Autodesk Fusion 360 part; units mm, degrees
note: some values were not read from the file. Set by a fixed rule: which sketch regions a step uses.
(part 9 of 10)
  spline S50 degree 5 poles (-7.6003, -14.0796) (-7.5986, -14.0783) (-7.5952, -14.0758) (-7.5901, -14.0719) (-7.5833, -14.0668) (-7.5749, -14.0604) (-7.5665, -14.0541) (-7.5581, -14.0477) (-7.5497, -14.0413) (-7.5414, -14.035) (-7.5331, -14.0286) (-7.5248, -14.0222) (-7.5166, -14.0159) (-7.5084, -14.0095) (-7.5002, -14.0032) (-7.4921, -13.9968) (-7.484, -13.9905) (-7.4759, -13.9841) (-7.4679, -13.9778) (-7.4599, -13.9714) (-7.4519, -13.9651) (-7.4439, -13.9588) (-7.436, -13.9525) (-7.4281, -13.9461) (-7.4203, -13.9398) (-7.4124, -13.9335) (-7.4046, -13.9272) (-7.3969, -13.9209) (-7.3892, -13.9146) (-7.3815, -13.9083) (-7.3738, -13.902) (-7.3662, -13.8958) (-7.3586, -13.8895) (-7.351, -13.8832) (-7.3435, -13.8769) (-7.336, -13.8707) (-7.3285, -13.8644) (-7.321, -13.8582) (-7.3136, -13.8519) (-7.3063, -13.8457) (-7.2989, -13.8395) (-7.2916, -13.8333) (-7.2843, -13.827) (-7.2771, -13.8208) (-7.2699, -13.8146) (-7.2627, -13.8084) (-7.2555, -13.8023) (-7.2484, -13.7961) (-7.2413, -13.7899) (-7.2343, -13.7837) (-7.2272, -13.7776) (-7.2203, -13.7714) (-7.2133, -13.7653) (-7.2064, -13.7592) (-7.1995, -13.753) (-7.1926, -13.7469) (-7.1858, -13.7408) (-7.179, -13.7347) (-7.1723, -13.7286) (-7.1655, -13.7226) (-7.1588, -13.7165) (-7.1522, -13.7104) (-7.1455, -13.7044) (-7.1389, -13.6983) (-7.1324, -13.6923) (-7.1259, -13.6863) (-7.1194, -13.6803) (-7.1129, -13.6743) (-7.1065, -13.6683) (-7.1001, -13.6623) (-7.0937, -13.6563) (-7.0874, -13.6504) (-7.0811, -13.6444) (-7.0748, -13.6385) (-7.0686, -13.6325) (-7.0624, -13.6266) (-7.0562, -13.6207) (-7.0501, -13.6148) (-7.044, -13.6089) (-7.0379, -13.6031) (-7.0319, -13.5972) (-7.0259, -13.5914) (-7.02, -13.5855) (-7.014, -13.5797) (-7.0081, -13.5739) (-7.0023, -13.5681) (-6.9965, -13.5624) (-6.9907, -13.5566) (-6.9849, -13.5508) (-6.9792, -13.5451) (-6.9735, -13.5394) (-6.9678, -13.5337) (-6.9622, -13.528) (-6.9566, -13.5223) (-6.9511, -13.5166) (-6.9455, -13.511) (-6.94, -13.5053) (-6.9346, -13.4997) (-6.9292, -13.4941) (-6.9238, -13.4885) (-6.9184, -13.4829) (-6.9131, -13.4774) (-6.9078, -13.4718) (-6.9026, -13.4663) (-6.8974, -13.4608) (-6.8922, -13.4553) (-6.8871, -13.4498) (-6.8819, -13.4444) (-6.8769, -13.4389) (-6.8718, -13.4335) (-6.8668, -13.4281) (-6.8618, -13.4227) (-6.8569, -13.4173) (-6.852, -13.412) (-6.8471, -13.4066) (-6.8423, -13.4013) (-6.8375, -13.396) (-6.8327, -13.3907) (-6.828, -13.3855) (-6.8233, -13.3802) (-6.8187, -13.375) (-6.814, -13.3698) (-6.8094, -13.3646) (-6.8049, -13.3595) (-6.8004, -13.3543) (-6.7959, -13.3492) (-6.7914, -13.3441) (-6.787, -13.339) (-6.7826, -13.334) (-6.7783, -13.329) (-6.774, -13.3239) (-6.7697, -13.319) (-6.7655, -13.314) (-6.7613, -13.309) (-6.7571, -13.3041) (-6.753, -13.2992) (-6.7489, -13.2944) (-6.7448, -13.2895) (-6.7408, -13.2847) (-6.7368, -13.2799) (-6.7328, -13.2751) (-6.7289, -13.2703) (-6.725, -13.2656) (-6.7212, -13.2609) (-6.7174, -13.2562) (-6.7136, -13.2516) (-6.7098, -13.2469) (-6.7061, -13.2423) (-6.7025, -13.2378) (-6.6988, -13.2332) (-6.6952, -13.2287) (-6.6917, -13.2242) (-6.6881, -13.2197) (-6.6846, -13.2153) (-6.6812, -13.2109) (-6.6778, -13.2065) (-6.6744, -13.2022) (-6.671, -13.1978) (-6.6677, -13.1935) (-6.6644, -13.1893) (-6.6612, -13.185) (-6.658, -13.1808) (-6.6548, -13.1767) (-6.6517, -13.1725) (-6.6486, -13.1684) (-6.6455, -13.1643) (-6.6425, -13.1603) (-6.6395, -13.1563) (-6.6366, -13.1523) (-6.6337, -13.1483) (-6.6308, -13.1444) (-6.628, -13.1405) (-6.6252, -13.1367) (-6.6224, -13.1328) (-6.6197, -13.1291) (-6.617, -13.1253) (-6.6143, -13.1216) (-6.6117, -13.1179) (-6.6091, -13.1143) (-6.6065, -13.1107) (-6.604, -13.1071) (-6.6016, -13.1036) (-6.5991, -13.1001) (-6.5967, -13.0966) (-6.5944, -13.0932) (-6.592, -13.0898) (-6.5897, -13.0865) (-6.5875, -13.0832) (-6.5853, -13.0799) (-6.5831, -13.0767) (-6.581, -13.0735) (-6.5788, -13.0703) (-6.5768, -13.0672) (-6.5747, -13.0642) (-6.5728, -13.0612) (-6.5708, -13.0582) (-6.5689, -13.0553) (-6.567, -13.0524) (-6.5651, -13.0495) (-6.5633, -13.0467) (-6.5616, -13.044) (-6.5598, -13.0413) (-6.5581, -13.0386) (-6.5565, -13.036) (-6.5549, -13.0334) (-6.5533, -13.0309) (-6.5517, -13.0284) (-6.5502, -13.026) (-6.5488, -13.0236) (-6.5473, -13.0213) (-6.5459, -13.019) (-6.5446, -13.0168) (-6.5433, -13.0146) (-6.542, -13.0125) (-6.5407, -13.0104) (-6.5395, -13.0084) (-6.5384, -13.0064) (-6.5372, -13.0045) (-6.5361, -13.0027) (-6.5351, -13.0009) (-6.5341, -12.9991) (-6.5331, -12.9974) (-6.5321, -12.9958) (-6.5312, -12.9942) (-6.5304, -12.9927) (-6.5295, -12.9913) (-6.5288, -12.9899) (-6.528, -12.9885) (-6.5273, -12.9873) (-6.5266, -12.986) (-6.526, -12.9849) (-6.5254, -12.9838) (-6.5248, -12.9828) (-6.5243, -12.9818) (-6.5238, -12.9809) (-6.5234, -12.9801) (-6.523, -12.9794) (-6.5226, -12.9787) (-6.5223, -12.9781) (-6.522, -12.9775) (-6.5218, -12.977) (-6.5216, -12.9767) (-6.5215, -12.9765) (-6.5214, -12.9764) (-6.5214, -12.9763) knots -1 -1 -1 -1 -1 -1 -0.99583333 -0.99166667 -0.9875 -0.98333333 -0.97916667 -0.975 -0.97083333 -0.96666667 -0.9625 -0.95833333 -0.95416667 -0.95 -0.94583333 -0.94166667 -0.9375 -0.93333333 -0.92916667 -0.925 -0.92083333 -0.91666667 -0.9125 -0.90833333 -0.90416667 -0.9 -0.89583333 -0.89166667 -0.8875 -0.88333333 -0.87916667 -0.875 -0.87083333 -0.86666667 -0.8625 -0.85833333 -0.85416667 -0.85 -0.84583333 -0.84166667 -0.8375 -0.83333333 -0.82916667 -0.825 -0.82083333 -0.81666667 -0.8125 -0.80833333 -0.80416667 -0.8 -0.79583333 -0.79166667 -0.7875 -0.78333333 -0.77916667 -0.775 -0.77083333 -0.76666667 -0.7625 -0.75833333 -0.75416667 -0.75 -0.74583333 -0.74166667 -0.7375 -0.73333333 -0.72916667 -0.725 -0.72083333 -0.71666667 -0.7125 -0.70833333 -0.70416667 -0.7 -0.69583333 -0.69166667 -0.6875 -0.68333333 -0.67916667 -0.675 -0.67083333 -0.66666667 -0.6625 -0.65833333 -0.65416667 -0.65 -0.64583333 -0.64166667 -0.6375 -0.63333333 -0.62916667 -0.625 -0.62083333 -0.61666667 -0.6125 -0.60833333 -0.60416667 -0.6 -0.59583333 -0.59166667 -0.5875 -0.58333333 -0.57916667 -0.575 -0.57083333 -0.56666667 -0.5625 -0.55833333 -0.55416667 -0.55 -0.54583333 -0.54166667 -0.5375 -0.53333333 -0.52916667 -0.525 -0.52083333 -0.51666667 -0.5125 -0.50833333 -0.50416667 -0.5 -0.49583333 -0.49166667 -0.4875 -0.48333333 -0.47916667 -0.475 -0.47083333 -0.46666667 -0.4625 -0.45833333 -0.45416667 -0.45 -0.44583333 -0.44166667 -0.4375 -0.43333333 -0.42916667 -0.425 -0.42083333 -0.41666667 -0.4125 -0.40833333 -0.40416667 -0.4 -0.39583333 -0.39166667 -0.3875 -0.38333333 -0.37916667 -0.375 -0.37083333 -0.36666667 -0.3625 -0.35833333 -0.35416667 -0.35 -0.34583333 -0.34166667 -0.3375 -0.33333333 -0.32916667 -0.325 -0.32083333 -0.31666667 -0.3125 -0.30833333 -0.30416667 -0.3 -0.29583333 -0.29166667 -0.2875 -0.28333333 -0.27916667 -0.275 -0.27083333 -0.26666667 -0.2625 -0.25833333 -0.25416667 -0.25 -0.24583333 -0.24166667 -0.2375 -0.23333333 -0.22916667 -0.225 -0.22083333 -0.21666667 -0.2125 -0.20833333 -0.20416667 -0.2 -0.19583333 -0.19166667 -0.1875 -0.18333333 -0.17916667 -0.175 -0.17083333 -0.16666667 -0.1625 -0.15833333 -0.15416667 -0.15 -0.14583333 -0.14166667 -0.1375 -0.13333333 -0.12916667 -0.125 -0.12083333 -0.11666667 -0.1125 -0.10833333 -0.10416667 -0.1 -0.09583333 -0.09166667 -0.0875 -0.08333333 -0.07916667 -0.075 -0.07083333 -0.06666667 -0.0625 -0.05833333 -0.05416667 -0.05 -0.04583333 -0.04166667 -0.0375 -0.03333333 -0.02916667 -0.025 -0.02083333 -0.01666667 -0.0125 -0.00833333 -0.00416667 0 0 0 0 0 0
  line L101 (-12.9026, 6.6646) -> (-12.9032, 6.6649)
  spline S51 degree 5 poles (-5.2796, -13.5292) (-5.2796, -13.5293) (-5.2797, -13.5294) (-5.2798, -13.5296) (-5.2799, -13.53) (-5.2801, -13.5305) (-5.2803, -13.531) (-5.2805, -13.5317) (-5.2808, -13.5324) (-5.2811, -13.5332) (-5.2814, -13.5341) (-5.2818, -13.5351) (-5.2821, -13.5361) (-5.2825, -13.5372) (-5.2829, -13.5383) (-5.2833, -13.5396) (-5.2838, -13.5409) (-5.2843, -13.5423) (-5.2848, -13.5437) (-5.2853, -13.5452) (-5.2858, -13.5468) (-5.2863, -13.5485) (-5.2869, -13.5502) (-5.2875, -13.552) (-5.2881, -13.5539) (-5.2887, -13.5558) (-5.2893, -13.5578) (-5.29, -13.5598) (-5.2907, -13.5619) (-5.2913, -13.5641) (-5.292, -13.5664) (-5.2927, -13.5687) (-5.2935, -13.5711) (-5.2942, -13.5735) (-5.2949, -13.576) (-5.2957, -13.5786) (-5.2965, -13.5812) (-5.2972, -13.5839) (-5.298, -13.5866) (-5.2988, -13.5894) (-5.2997, -13.5923) (-5.3005, -13.5952) (-5.3013, -13.5982) (-5.3022, -13.6012) (-5.303, -13.6043) (-5.3039, -13.6075) (-5.3047, -13.6107) (-5.3056, -13.614) (-5.3065, -13.6173) (-5.3074, -13.6207) (-5.3083, -13.6241) (-5.3092, -13.6276) (-5.3101, -13.6312) (-5.3111, -13.6348) (-5.312, -13.6385) (-5.3129, -13.6422) (-5.3138, -13.646) (-5.3148, -13.6498) (-5.3157, -13.6537) (-5.3167, -13.6576) (-5.3176, -13.6616) (-5.3186, -13.6657) (-5.3196, -13.6698) (-5.3205, -13.6739) (-5.3215, -13.6781) (-5.3225, -13.6824) (-5.3235, -13.6867) (-5.3244, -13.691) (-5.3254, -13.6954) (-5.3264, -13.6999) (-5.3274, -13.7044) (-5.3284, -13.709) (-5.3293, -13.7136) (-5.3303, -13.7183) (-5.3313, -13.723) (-5.3323, -13.7277) (-5.3333, -13.7325) (-5.3343, -13.7374) (-5.3353, -13.7423) (-5.3363, -13.7473) (-5.3372, -13.7523) (-5.3382, -13.7573) (-5.3392, -13.7624) (-5.3402, -13.7676) (-5.3412, -13.7728) (-5.3422, -13.778) (-5.3431, -13.7833) (-5.3441, -13.7886) (-5.3451, -13.794) (-5.3461, -13.7994) (-5.347, -13.8049) (-5.348, -13.8104) (-5.3489, -13.816) (-5.3499, -13.8216) (-5.3509, -13.8273) (-5.3518, -13.833) (-5.3528, -13.8387) (-5.3537, -13.8445) (-5.3546, -13.8503) (-5.3556, -13.8562) (-5.3565, -13.8621) (-5.3574, -13.8681) (-5.3583, -13.8741) (-5.3593, -13.8801) (-5.3602, -13.8862) (-5.3611, -13.8924) (-5.362, -13.8986) (-5.3629, -13.9048) (-5.3638, -13.911) (-5.3646, -13.9173) (-5.3655, -13.9237) (-5.3664, -13.9301) (-5.3672, -13.9365) (-5.3681, -13.943) (-5.3689, -13.9495) (-5.3698, -13.9561) (-5.3706, -13.9627) (-5.3714, -13.9693) (-5.3723, -13.976) (-5.3731, -13.9827) (-5.3739, -13.9895) (-5.3747, -13.9963) (-5.3755, -14.0031) (-5.3762, -14.01) (-5.377, -14.0169) (-5.3778, -14.0238) (-5.3785, -14.0308) (-5.3793, -14.0379) (-5.38, -14.0449) (-5.3807, -14.0521) (-5.3814, -14.0592) (-5.3821, -14.0664) (-5.3828, -14.0736) (-5.3835, -14.0809) (-5.3842, -14.0882) (-5.3849, -14.0955) (-5.3855, -14.1029) (-5.3862, -14.1103) (-5.3868, -14.1178) (-5.3874, -14.1253) (-5.3881, -14.1328) (-5.3887, -14.1403) (-5.3893, -14.1479) (-5.3899, -14.1556) (-5.3904, -14.1632) (-5.391, -14.171) (-5.3915, -14.1787) (-5.3921, -14.1865) (-5.3926, -14.1943) (-5.3931, -14.2021) (-5.3936, -14.21) (-5.3941, -14.2179) (-5.3946, -14.2259) (-5.3951, -14.2339) (-5.3955, -14.2419) (-5.396, -14.25) (-5.3964, -14.2581) (-5.3968, -14.2662) (-5.3973, -14.2744) (-5.3976, -14.2826) (-5.398, -14.2908) (-5.3984, -14.2991) (-5.3988, -14.3074) (-5.3991, -14.3157) (-5.3994, -14.3241) (-5.3998, -14.3325) (-5.4001, -14.3409) (-5.4003, -14.3493) (-5.4006, -14.3578) (-5.4009, -14.3664) (-5.4011, -14.3749) (-5.4014, -14.3835) (-5.4016, -14.3922) (-5.4018, -14.4008) (-5.402, -14.4095) (-5.4022, -14.4182) (-5.4023, -14.427) (-5.4025, -14.4358) (-5.4026, -14.4446) (-5.4028, -14.4535) (-5.4029, -14.4623) (-5.403, -14.4712) (-5.403, -14.4802) (-5.4031, -14.4892) (-5.4031, -14.4982) (-5.4032, -14.5072) (-5.4032, -14.5163) (-5.4032, -14.5254) (-5.4032, -14.5345) (-5.4032, -14.5437) (-5.4031, -14.5528) (-5.4031, -14.5621) (-5.403, -14.5713) (-5.4029, -14.5806) (-5.4028, -14.5899) (-5.4027, -14.5992) (-5.4025, -14.6086) (-5.4024, -14.618) (-5.4022, -14.6274) (-5.402, -14.6369) (-5.4018, -14.6464) (-5.4016, -14.6559) (-5.4013, -14.6654) (-5.4011, -14.675) (-5.4008, -14.6846) (-5.4005, -14.6942) (-5.4002, -14.7038) (-5.3999, -14.7135) (-5.3996, -14.7232) (-5.3992, -14.733) (-5.3988, -14.7427) (-5.3985, -14.7525) (-5.3981, -14.7624) (-5.3976, -14.7722) (-5.3972, -14.7821) (-5.3967, -14.792) (-5.3963, -14.8019) (-5.3958, -14.8119) (-5.3953, -14.8218) (-5.3947, -14.8319) (-5.3942, -14.8419) (-5.3936, -14.852) (-5.393, -14.862) (-5.3924, -14.8722) (-5.3918, -14.8823) (-5.3912, -14.8925) (-5.3905, -14.9027) (-5.3899, -14.9129) (-5.3892, -14.9231) (-5.3885, -14.9334) (-5.3877, -14.9437) (-5.387, -14.954) (-5.3862, -14.9644) (-5.3854, -14.9747) (-5.3846, -14.9851) (-5.3838, -14.9956) (-5.383, -15.006) (-5.3821, -15.0165) (-5.3813, -15.027) (-5.3804, -15.0375) (-5.3794, -15.0481) (-5.3787, -15.0565) (-5.3781, -15.0629) (-5.3777, -15.0671) (-5.3776, -15.0692) knots 0 0 0 0 0 0 0.00416667 0.00833333 0.0125 0.01666667 0.02083333 0.025 0.02916667 0.03333333 0.0375 0.04166667 0.04583333 0.05 0.05416667 0.05833333 0.0625 0.06666667 0.07083333 0.075 0.07916667 0.08333333 0.0875 0.09166667 0.09583333 0.1 0.10416667 0.10833333 0.1125 0.11666667 0.12083333 0.125 0.12916667 0.13333333 0.1375 0.14166667 0.14583333 0.15 0.15416667 0.15833333 0.1625 0.16666667 0.17083333 0.175 0.17916667 0.18333333 0.1875 0.19166667 0.19583333 0.2 0.20416667 0.20833333 0.2125 0.21666667 0.22083333 0.225 0.22916667 0.23333333 0.2375 0.24166667 0.24583333 0.25 0.25416667 0.25833333 0.2625 0.26666667 0.27083333 0.275 0.27916667 0.28333333 0.2875 0.29166667 0.29583333 0.3 0.30416667 0.30833333 0.3125 0.31666667 0.32083333 0.325 0.32916667 0.33333333 0.3375 0.34166667 0.34583333 0.35 0.35416667 0.35833333 0.3625 0.36666667 0.37083333 0.375 0.37916667 0.38333333 0.3875 0.39166667 0.39583333 0.4 0.40416667 0.40833333 0.4125 0.41666667 0.42083333 0.425 0.42916667 0.43333333 0.4375 0.44166667 0.44583333 0.45 0.45416667 0.45833333 0.4625 0.46666667 0.47083333 0.475 0.47916667 0.48333333 0.4875 0.49166667 0.49583333 0.5 0.50416667 0.50833333 0.5125 0.51666667 0.52083333 0.525 0.52916667 0.53333333 0.5375 0.54166667 0.54583333 0.55 0.55416667 0.55833333 0.5625 0.56666667 0.57083333 0.575 0.57916667 0.58333333 0.5875 0.59166667 0.59583333 0.6 0.60416667 0.60833333 0.6125 0.61666667 0.62083333 0.625 0.62916667 0.63333333 0.6375 0.64166667 0.64583333 0.65 0.65416667 0.65833333 0.6625 0.66666667 0.67083333 0.675 0.67916667 0.68333333 0.6875 0.69166667 0.69583333 0.7 0.70416667 0.70833333 0.7125 0.71666667 0.72083333 0.725 0.72916667 0.73333333 0.7375 0.74166667 0.74583333 0.75 0.75416667 0.75833333 0.7625 0.76666667 0.77083333 0.775 0.77916667 0.78333333 0.7875 0.79166667 0.79583333 0.8 0.80416667 0.80833333 0.8125 0.81666667 0.82083333 0.825 0.82916667 0.83333333 0.8375 0.84166667 0.84583333 0.85 0.85416667 0.85833333 0.8625 0.86666667 0.87083333 0.875 0.87916667 0.88333333 0.8875 0.89166667 0.89583333 0.9 0.90416667 0.90833333 0.9125 0.91666667 0.92083333 0.925 0.92916667 0.93333333 0.9375 0.94166667 0.94583333 0.95 0.95416667 0.95833333 0.9625 0.96666667 0.97083333 0.975 0.97916667 0.98333333 0.9875 0.99166667 0.99583333 1 1 1 1 1 1
  spline S52 degree 5 poles (-14.007, 3.8365) (-14.007, 3.8365) (-14.0072, 3.8366) (-14.0074, 3.8366) (-14.0077, 3.8367) (-14.0083, 3.8369) (-14.0089, 3.837) (-14.0095, 3.8372) (-14.0103, 3.8374) (-14.0111, 3.8376) (-14.012, 3.8378) (-14.013, 3.838) (-14.0141, 3.8383) (-14.0152, 3.8386) (-14.0164, 3.8388) (-14.0177, 3.8391) (-14.019, 3.8394) (-14.0204, 3.8398) (-14.0219, 3.8401) (-14.0235, 3.8405) (-14.0251, 3.8408) (-14.0268, 3.8412) (-14.0286, 3.8416) (-14.0305, 3.842) (-14.0324, 3.8424) (-14.0343, 3.8428) (-14.0364, 3.8432) (-14.0385, 3.8436) (-14.0407, 3.8441) (-14.0429, 3.8445) (-14.0452, 3.845) (-14.0476, 3.8454) (-14.05, 3.8459) (-14.0525, 3.8464) (-14.0551, 3.8469) (-14.0577, 3.8473) (-14.0604, 3.8478) (-14.0632, 3.8483) (-14.066, 3.8488) (-14.0688, 3.8493) (-14.0718, 3.8498) (-14.0748, 3.8504) (-14.0778, 3.8509) (-14.0809, 3.8514) (-14.0841, 3.8519) (-14.0873, 3.8525) (-14.0906, 3.853) (-14.094, 3.8535) (-14.0974, 3.854) (-14.1009, 3.8546) (-14.1044, 3.8551) (-14.1079, 3.8557) (-14.1116, 3.8562) (-14.1153, 3.8567) (-14.119, 3.8573) (-14.1228, 3.8578) (-14.1267, 3.8583) (-14.1306, 3.8589) (-14.1345, 3.8594) (-14.1386, 3.86) (-14.1426, 3.8605) (-14.1467, 3.861) (-14.1509, 3.8615) (-14.1552, 3.8621) (-14.1594, 3.8626) (-14.1638, 3.8631) (-14.1682, 3.8636) (-14.1726, 3.8642) (-14.1771, 3.8647) (-14.1816, 3.8652) (-14.1862, 3.8657) (-14.1908, 3.8662) (-14.1955, 3.8667) (-14.2003, 3.8672) (-14.2051, 3.8677) (-14.2099, 3.8682) (-14.2148, 3.8686) (-14.2197, 3.8691) (-14.2247, 3.8696) (-14.2297, 3.87) (-14.2348, 3.8705) (-14.2399, 3.871) (-14.2451, 3.8714) (-14.2503, 3.8718) (-14.2556, 3.8723) (-14.2609, 3.8727) (-14.2663, 3.8731) (-14.2717, 3.8735) (-14.2771, 3.8739) (-14.2826, 3.8743) (-14.2882, 3.8747) (-14.2938, 3.8751) (-14.2994, 3.8755) (-14.3051, 3.8758) (-14.3108, 3.8762) (-14.3166, 3.8766) (-14.3224, 3.8769) (-14.3283, 3.8772) (-14.3342, 3.8776) (-14.3401, 3.8779) (-14.3461, 3.8782) (-14.3521, 3.8785) (-14.3582, 3.8788) (-14.3643, 3.879) (-14.3705, 3.8793) (-14.3767, 3.8796) (-14.3829, 3.8798) (-14.3892, 3.88) (-14.3955, 3.8803) (-14.4019, 3.8805) (-14.4083, 3.8807) (-14.4147, 3.8809) (-14.4212, 3.8811) (-14.4277, 3.8812) (-14.4343, 3.8814) (-14.4409, 3.8816) (-14.4476, 3.8817) (-14.4542, 3.8818) (-14.461, 3.8819) (-14.4677, 3.882) (-14.4745, 3.8821) (-14.4814, 3.8822) (-14.4883, 3.8823) (-14.4952, 3.8823) (-14.5021, 3.8824) (-14.5091, 3.8824) (-14.5162, 3.8824) (-14.5233, 3.8824) (-14.5304, 3.8824) (-14.5375, 3.8824) (-14.5447, 3.8824) (-14.5519, 3.8823) (-14.5592, 3.8823) (-14.5665, 3.8822) (-14.5738, 3.8821) (-14.5812, 3.882) (-14.5886, 3.8819) (-14.596, 3.8817) (-14.6035, 3.8816) (-14.611, 3.8814) (-14.6186, 3.8813) (-14.6261, 3.8811) (-14.6338, 3.8809) (-14.6414, 3.8807) (-14.6491, 3.8804) (-14.6568, 3.8802) (-14.6646, 3.8799) (-14.6724, 3.8797) (-14.6802, 3.8794) (-14.6881, 3.8791) (-14.696, 3.8787) (-14.7039, 3.8784) (-14.7119, 3.878) (-14.7199, 3.8777) (-14.7279, 3.8773) (-14.7359, 3.8769) (-14.744, 3.8765) (-14.7522, 3.8761) (-14.7603, 3.8756) (-14.7685, 3.8751) (-14.7768, 3.8747) (-14.785, 3.8742) (-14.7933, 3.8737) (-14.8016, 3.8731) (-14.81, 3.8726) (-14.8184, 3.872) (-14.8268, 3.8714) (-14.8352, 3.8708) (-14.8437, 3.8702) (-14.8522, 3.8696) (-14.8608, 3.869) (-14.8693, 3.8683) (-14.8779, 3.8676) (-14.8866, 3.8669) (-14.8952, 3.8662) (-14.9039, 3.8655) (-14.9127, 3.8647) (-14.9214, 3.8639) (-14.9302, 3.8632) (-14.939, 3.8624) (-14.9479, 3.8615) (-14.9567, 3.8607) (-14.9656, 3.8598) (-14.9746, 3.859) (-14.9835, 3.8581) (-14.9925, 3.8572) (-15.0015, 3.8562) (-15.0106, 3.8553) (-15.0197, 3.8543) (-15.0288, 3.8533) (-15.0379, 3.8523) (-15.0471, 3.8513) (-15.0563, 3.8503) (-15.0655, 3.8492) (-15.0747, 3.8481) (-15.084, 3.847) (-15.0933, 3.8459) (-15.1026, 3.8448) (-15.112, 3.8436) (-15.1214, 3.8424) (-15.1308, 3.8412) (-15.1402, 3.84) (-15.1497, 3.8388) (-15.1591, 3.8375) (-15.1687, 3.8363) (-15.1782, 3.835) (-15.1878, 3.8337) (-15.1974, 3.8323) (-15.207, 3.831) (-15.2166, 3.8296) (-15.2263, 3.8282) (-15.236, 3.8268) (-15.2457, 3.8254) (-15.2555, 3.8239) (-15.2653, 3.8225) (-15.2751, 3.821) (-15.2849, 3.8195) (-15.2947, 3.8179) (-15.3046, 3.8164) (-15.3145, 3.8148) (-15.3244, 3.8132) (-15.3344, 3.8116) (-15.3444, 3.81) (-15.3544, 3.8083) (-15.3644, 3.8067) (-15.3744, 3.805) (-15.3845, 3.8033) (-15.3946, 3.8015) (-15.4047, 3.7998) (-15.4148, 3.798) (-15.425, 3.7962) (-15.4352, 3.7944) (-15.4454, 3.7925) (-15.4556, 3.7907) (-15.4659, 3.7888) (-15.4762, 3.7869) (-15.4865, 3.7849) (-15.4968, 3.783) (-15.5072, 3.781) (-15.5175, 3.779) (-15.5279, 3.777) (-15.5363, 3.7754) (-15.5425, 3.7742) (-15.5467, 3.7733) (-15.5488, 3.7729) knots 0 0 0 0 0 0 0.00416667 0.00833333 0.0125 0.01666667 0.02083333 0.025 0.02916667 0.03333333 0.0375 0.04166667 0.04583333 0.05 0.05416667 0.05833333 0.0625 0.06666667 0.07083333 0.075 0.07916667 0.08333333 0.0875 0.09166667 0.09583333 0.1 0.10416667 0.10833333 0.1125 0.11666667 0.12083333 0.125 0.12916667 0.13333333 0.1375 0.14166667 0.14583333 0.15 0.15416667 0.15833333 0.1625 0.16666667 0.17083333 0.175 0.17916667 0.18333333 0.1875 0.19166667 0.19583333 0.2 0.20416667 0.20833333 0.2125 0.21666667 0.22083333 0.225 0.22916667 0.23333333 0.2375 0.24166667 0.24583333 0.25 0.25416667 0.25833333 0.2625 0.26666667 0.27083333 0.275 0.27916667 0.28333333 0.2875 0.29166667 0.29583333 0.3 0.30416667 0.30833333 0.3125 0.31666667 0.32083333 0.325 0.32916667 0.33333333 0.3375 0.34166667 0.34583333 0.35 0.35416667 0.35833333 0.3625 0.36666667 0.37083333 0.375 0.37916667 0.38333333 0.3875 0.39166667 0.39583333 0.4 0.40416667 0.40833333 0.4125 0.41666667 0.42083333 0.425 0.42916667 0.43333333 0.4375 0.44166667 0.44583333 0.45 0.45416667 0.45833333 0.4625 0.46666667 0.47083333 0.475 0.47916667 0.48333333 0.4875 0.49166667 0.49583333 0.5 0.50416667 0.50833333 0.5125 0.51666667 0.52083333 0.525 0.52916667 0.53333333 0.5375 0.54166667 0.54583333 0.55 0.55416667 0.55833333 0.5625 0.56666667 0.57083333 0.575 0.57916667 0.58333333 0.5875 0.59166667 0.59583333 0.6 0.60416667 0.60833333 0.6125 0.61666667 0.62083333 0.625 0.62916667 0.63333333 0.6375 0.64166667 0.64583333 0.65 0.65416667 0.65833333 0.6625 0.66666667 0.67083333 0.675 0.67916667 0.68333333 0.6875 0.69166667 0.69583333 0.7 0.70416667 0.70833333 0.7125 0.71666667 0.72083333 0.725 0.72916667 0.73333333 0.7375 0.74166667 0.74583333 0.75 0.75416667 0.75833333 0.7625 0.76666667 0.77083333 0.775 0.77916667 0.78333333 0.7875 0.79166667 0.79583333 0.8 0.80416667 0.80833333 0.8125 0.81666667 0.82083333 0.825 0.82916667 0.83333333 0.8375 0.84166667 0.84583333 0.85 0.85416667 0.85833333 0.8625 0.86666667 0.87083333 0.875 0.87916667 0.88333333 0.8875 0.89166667 0.89583333 0.9 0.90416667 0.90833333 0.9125 0.91666667 0.92083333 0.925 0.92916667 0.93333333 0.9375 0.94166667 0.94583333 0.95 0.95416667 0.95833333 0.9625 0.96666667 0.97083333 0.975 0.97916667 0.98333333 0.9875 0.99166667 0.99583333 1 1 1 1 1 1
  line L102 (-14.4979, 0.8404) -> (-14.4985, 0.8405)
  line L103 (-0.6796, -14.5069) -> (-0.6796, -14.5063)
  line L104 (-13.727, 0.7957) -> (-14.4979, 0.8404)
  arc A60 (-13.5924, 2.0756) -> (-13.727, 0.7957) centre (0, 0) ccw
  spline S53 degree 5 poles (-15.7391, 2.8775) (-15.7374, 2.8763) (-15.7339, 2.8738) (-15.7287, 2.8702) (-15.7217, 2.8653) (-15.713, 2.8592) (-15.7044, 2.8532) (-15.6957, 2.8472) (-15.6871, 2.8412) (-15.6785, 2.8353) (-15.6698, 2.8293) (-15.6612, 2.8234) (-15.6526, 2.8176) (-15.6441, 2.8117) (-15.6355, 2.8059) (-15.6269, 2.8002) (-15.6184, 2.7944) (-15.6099, 2.7887) (-15.6014, 2.783) (-15.5929, 2.7773) (-15.5844, 2.7717) (-15.5759, 2.7661) (-15.5674, 2.7605) (-15.559, 2.755) (-15.5505, 2.7494) (-15.5421, 2.744) (-15.5337, 2.7385) (-15.5253, 2.7331) (-15.517, 2.7277) (-15.5086, 2.7223) (-15.5002, 2.7169) (-15.4919, 2.7116) (-15.4836, 2.7063) (-15.4753, 2.7011) (-15.467, 2.6958) (-15.4587, 2.6906) (-15.4505, 2.6855) (-15.4422, 2.6803) (-15.434, 2.6752) (-15.4258, 2.6701) (-15.4176, 2.665) (-15.4094, 2.66) (-15.4013, 2.655) (-15.3931, 2.65) (-15.385, 2.6451) (-15.3769, 2.6402) (-15.3688, 2.6353) (-15.3607, 2.6304) (-15.3527, 2.6256) (-15.3446, 2.6208) (-15.3366, 2.616) (-15.3286, 2.6113) (-15.3206, 2.6065) (-15.3126, 2.6019) (-15.3047, 2.5972) (-15.2968, 2.5926) (-15.2888, 2.588) (-15.2809, 2.5834) (-15.2731, 2.5788) (-15.2652, 2.5743) (-15.2574, 2.5698) (-15.2495, 2.5654) (-15.2417, 2.5609) (-15.2339, 2.5565) (-15.2262, 2.5522) (-15.2184, 2.5478) (-15.2107, 2.5435) (-15.203, 2.5392) (-15.1953, 2.5349) (-15.1876, 2.5307) (-15.18, 2.5265) (-15.1724, 2.5223) (-15.1648, 2.5182) (-15.1572, 2.514) (-15.1496, 2.5099) (-15.1421, 2.5059) (-15.1346, 2.5018) (-15.1271, 2.4978) (-15.1196, 2.4939) (-15.1121, 2.4899) (-15.1047, 2.486) (-15.0973, 2.4821) (-15.0899, 2.4782) (-15.0825, 2.4744) (-15.0752, 2.4706) (-15.0679, 2.4668) (-15.0606, 2.463) (-15.0533, 2.4593) (-15.0461, 2.4556) (-15.0388, 2.4519) (-15.0316, 2.4483) (-15.0245, 2.4447) (-15.0173, 2.4411) (-15.0102, 2.4375) (-15.0031, 2.434) (-14.996, 2.4305) (-14.9889, 2.427) (-14.9819, 2.4236) (-14.9749, 2.4201) (-14.9679, 2.4167) (-14.9609, 2.4134) (-14.954, 2.41) (-14.9471, 2.4067) (-14.9402, 2.4034) (-14.9334, 2.4002) (-14.9266, 2.397) (-14.9198, 2.3938) (-14.913, 2.3906) (-14.9062, 2.3874) (-14.8995, 2.3843) (-14.8928, 2.3812) (-14.8862, 2.3782) (-14.8795, 2.3751) (-14.8729, 2.3721) (-14.8663, 2.3691) (-14.8598, 2.3662) (-14.8533, 2.3633) (-14.8468, 2.3604) (-14.8403, 2.3575) (-14.8339, 2.3546) (-14.8275, 2.3518) (-14.8211, 2.349) (-14.8148, 2.3463) (-14.8084, 2.3435) (-14.8022, 2.3408) (-14.7959, 2.3381) (-14.7897, 2.3355) (-14.7835, 2.3328) (-14.7773, 2.3302) (-14.7712, 2.3277) (-14.7651, 2.3251) (-14.759, 2.3226) (-14.753, 2.3201) (-14.747, 2.3176) (-14.741, 2.3152) (-14.7351, 2.3128) (-14.7292, 2.3104) (-14.7233, 2.308) (-14.7175, 2.3057) (-14.7117, 2.3034) (-14.7059, 2.3011) (-14.7002, 2.2988) (-14.6945, 2.2966) (-14.6888, 2.2944) (-14.6832, 2.2922) (-14.6776, 2.29) (-14.672, 2.2879) (-14.6665, 2.2858) (-14.661, 2.2837) (-14.6556, 2.2817) (-14.6502, 2.2796) (-14.6448, 2.2776) (-14.6395, 2.2757) (-14.6342, 2.2737) (-14.6289, 2.2718) (-14.6237, 2.2699) (-14.6185, 2.268) (-14.6133, 2.2662) (-14.6082, 2.2644) (-14.6032, 2.2626) (-14.5981, 2.2608) (-14.5932, 2.259) (-14.5882, 2.2573) (-14.5833, 2.2556) (-14.5784, 2.2539) (-14.5736, 2.2523) (-14.5688, 2.2507) (-14.5641, 2.2491) (-14.5594, 2.2475) (-14.5547, 2.2459) (-14.5501, 2.2444) (-14.5455, 2.2429) (-14.541, 2.2414) (-14.5365, 2.24) (-14.5321, 2.2386) (-14.5277, 2.2372) (-14.5233, 2.2358) (-14.519, 2.2344) (-14.5147, 2.2331) (-14.5105, 2.2318) (-14.5063, 2.2305) (-14.5022, 2.2292) (-14.4981, 2.228) (-14.4941, 2.2268) (-14.4901, 2.2256) (-14.4862, 2.2244) (-14.4823, 2.2233) (-14.4785, 2.2222) (-14.4747, 2.2211) (-14.4709, 2.22) (-14.4673, 2.2189) (-14.4636, 2.2179) (-14.46, 2.2169) (-14.4565, 2.2159) (-14.453, 2.2149) (-14.4496, 2.214) (-14.4462, 2.2131) (-14.4429, 2.2122) (-14.4396, 2.2113) (-14.4364, 2.2104) (-14.4332, 2.2096) (-14.4301, 2.2088) (-14.427, 2.208) (-14.424, 2.2072) (-14.4211, 2.2065) (-14.4182, 2.2058) (-14.4154, 2.2051) (-14.4126, 2.2044) (-14.4099, 2.2037) (-14.4072, 2.2031) (-14.4046, 2.2025) (-14.4021, 2.2018) (-14.3996, 2.2013) (-14.3972, 2.2007) (-14.3948, 2.2002) (-14.3925, 2.1996) (-14.3903, 2.1991) (-14.3882, 2.1986) (-14.386, 2.1982) (-14.384, 2.1977) (-14.382, 2.1973) (-14.3801, 2.1969) (-14.3783, 2.1965) (-14.3765, 2.1961) (-14.3748, 2.1958) (-14.3732, 2.1954) (-14.3716, 2.1951) (-14.3701, 2.1948) (-14.3687, 2.1945) (-14.3673, 2.1943) (-14.366, 2.194) (-14.3648, 2.1938) (-14.3637, 2.1936) (-14.3626, 2.1934) (-14.3616, 2.1932) (-14.3607, 2.193) (-14.3598, 2.1929) (-14.3591, 2.1928) (-14.3584, 2.1926) (-14.3578, 2.1925) (-14.3572, 2.1924) (-14.3569, 2.1924) (-14.3566, 2.1923) (-14.3565, 2.1923) (-14.3564, 2.1923) knots -1 -1 -1 -1 -1 -1 -0.99583333 -0.99166667 -0.9875 -0.98333333 -0.97916667 -0.975 -0.97083333 -0.96666667 -0.9625 -0.95833333 -0.95416667 -0.95 -0.94583333 -0.94166667 -0.9375 -0.93333333 -0.92916667 -0.925 -0.92083333 -0.91666667 -0.9125 -0.90833333 -0.90416667 -0.9 -0.89583333 -0.89166667 -0.8875 -0.88333333 -0.87916667 -0.875 -0.87083333 -0.86666667 -0.8625 -0.85833333 -0.85416667 -0.85 -0.84583333 -0.84166667 -0.8375 -0.83333333 -0.82916667 -0.825 -0.82083333 -0.81666667 -0.8125 -0.80833333 -0.80416667 -0.8 -0.79583333 -0.79166667 -0.7875 -0.78333333 -0.77916667 -0.775 -0.77083333 -0.76666667 -0.7625 -0.75833333 -0.75416667 -0.75 -0.74583333 -0.74166667 -0.7375 -0.73333333 -0.72916667 -0.725 -0.72083333 -0.71666667 -0.7125 -0.70833333 -0.70416667 -0.7 -0.69583333 -0.69166667 -0.6875 -0.68333333 -0.67916667 -0.675 -0.67083333 -0.66666667 -0.6625 -0.65833333 -0.65416667 -0.65 -0.64583333 -0.64166667 -0.6375 -0.63333333 -0.62916667 -0.625 -0.62083333 -0.61666667 -0.6125 -0.60833333 -0.60416667 -0.6 -0.59583333 -0.59166667 -0.5875 -0.58333333 -0.57916667 -0.575 -0.57083333 -0.56666667 -0.5625 -0.55833333 -0.55416667 -0.55 -0.54583333 -0.54166667 -0.5375 -0.53333333 -0.52916667 -0.525 -0.52083333 -0.51666667 -0.5125 -0.50833333 -0.50416667 -0.5 -0.49583333 -0.49166667 -0.4875 -0.48333333 -0.47916667 -0.475 -0.47083333 -0.46666667 -0.4625 -0.45833333 -0.45416667 -0.45 -0.44583333 -0.44166667 -0.4375 -0.43333333 -0.42916667 -0.425 -0.42083333 -0.41666667 -0.4125 -0.40833333 -0.40416667 -0.4 -0.39583333 -0.39166667 -0.3875 -0.38333333 -0.37916667 -0.375 -0.37083333 -0.36666667 -0.3625 -0.35833333 -0.35416667 -0.35 -0.34583333 -0.34166667 -0.3375 -0.33333333 -0.32916667 -0.325 -0.32083333 -0.31666667 -0.3125 -0.30833333 -0.30416667 -0.3 -0.29583333 -0.29166667 -0.2875 -0.28333333 -0.27916667 -0.275 -0.27083333 -0.26666667 -0.2625 -0.25833333 -0.25416667 -0.25 -0.24583333 -0.24166667 -0.2375 -0.23333333 -0.22916667 -0.225 -0.22083333 -0.21666667 -0.2125 -0.20833333 -0.20416667 -0.2 -0.19583333 -0.19166667 -0.1875 -0.18333333 -0.17916667 -0.175 -0.17083333 -0.16666667 -0.1625 -0.15833333 -0.15416667 -0.15 -0.14583333 -0.14166667 -0.1375 -0.13333333 -0.12916667 -0.125 -0.12083333 -0.11666667 -0.1125 -0.10833333 -0.10416667 -0.1 -0.09583333 -0.09166667 -0.0875 -0.08333333 -0.07916667 -0.075 -0.07083333 -0.06666667 -0.0625 -0.05833333 -0.05416667 -0.05 -0.04583333 -0.04166667 -0.0375 -0.03333333 -0.02916667 -0.025 -0.02083333 -0.01666667 -0.0125 -0.00833333 -0.00416667 0 0 0 0 0 0
  line L105 (-11.5731, -7.4247) -> (-12.223, -7.8417)
  line L106 (14.4985, 0.8405) -> (14.4979, 0.8404)
  arc A61 (-12.2165, -6.3102) -> (-11.5731, -7.4247) centre (0, 0) ccw
  arc A62 (12.6699, -9.771) -> (13.208, -9.0304) centre (0, 0) ccw
  arc A63 (10.3616, -12.1917) -> (11.0419, -11.5792) centre (0, 0) ccw
  arc A64 (12.2165, 6.3102) -> (11.5731, 7.4247) centre (0, 0) ccw
  spline S54 degree 5 poles (9.0768, -11.3369) (9.0769, -11.3369) (9.0769, -11.337) (9.0771, -11.3372) (9.0773, -11.3375) (9.0777, -11.3379) (9.0781, -11.3384) (9.0785, -11.3389) (9.079, -11.3395) (9.0796, -11.3402) (9.0802, -11.3409) (9.0808, -11.3417) (9.0815, -11.3425) (9.0823, -11.3434) (9.0831, -11.3443) (9.084, -11.3453) (9.0849, -11.3464) (9.0858, -11.3475) (9.0868, -11.3486) (9.0879, -11.3498) (9.089, -11.3511) (9.0902, -11.3524) (9.0914, -11.3537) (9.0926, -11.3551) (9.0939, -11.3566) (9.0953, -11.3581) (9.0967, -11.3596) (9.0982, -11.3612) (9.0997, -11.3628) (9.1012, -11.3645) (9.1028, -11.3662) (9.1045, -11.368) (9.1062, -11.3698) (9.1079, -11.3717) (9.1097, -11.3735) (9.1115, -11.3755) (9.1134, -11.3775) (9.1153, -11.3795) (9.1173, -11.3815) (9.1194, -11.3836) (9.1214, -11.3858) (9.1235, -11.388) (9.1257, -11.3902) (9.1279, -11.3924) (9.1302, -11.3947) (9.1325, -11.397) (9.1348, -11.3994) (9.1372, -11.4018) (9.1397, -11.4042) (9.1422, -11.4067) (9.1447, -11.4092) (9.1473, -11.4117) (9.1499, -11.4143) (9.1526, -11.4169) (9.1553, -11.4195) (9.158, -11.4222) (9.1608, -11.4249) (9.1637, -11.4276) (9.1666, -11.4304) (9.1695, -11.4332) (9.1725, -11.436) (9.1755, -11.4389) (9.1786, -11.4418) (9.1817, -11.4447) (9.1848, -11.4476) (9.188, -11.4506) (9.1913, -11.4536) (9.1946, -11.4566) (9.1979, -11.4597) (9.2013, -11.4627) (9.2047, -11.4658) (9.2081, -11.469) (9.2116, -11.4721) (9.2152, -11.4753) (9.2188, -11.4785) (9.2224, -11.4818) (9.2261, -11.485) (9.2298, -11.4883) (9.2335, -11.4916) (9.2373, -11.495) (9.2412, -11.4983) (9.2451, -11.5017) (9.249, -11.5051) (9.253, -11.5085) (9.257, -11.512) (9.261, -11.5154) (9.2651, -11.5189) (9.2692, -11.5224) (9.2734, -11.526) (9.2776, -11.5295) (9.2819, -11.5331) (9.2862, -11.5367) (9.2905, -11.5403) (9.2949, -11.544) (9.2993, -11.5476) (9.3038, -11.5513) (9.3083, -11.555) (9.3128, -11.5587) (9.3174, -11.5624) (9.322, -11.5662) (9.3267, -11.5699) (9.3314, -11.5737) (9.3361, -11.5775) (9.3409, -11.5813) (9.3457, -11.5852) (9.3506, -11.589) (9.3555, -11.5929) (9.3605, -11.5968) (9.3654, -11.6007) (9.3705, -11.6046) (9.3755, -11.6085) (9.3806, -11.6125) (9.3858, -11.6164) (9.3909, -11.6204) (9.3962, -11.6244) (9.4014, -11.6284) (9.4067, -11.6324) (9.412, -11.6365) (9.4174, -11.6405) (9.4228, -11.6446) (9.4283, -11.6486) (9.4338, -11.6527) (9.4393, -11.6568) (9.4449, -11.6609) (9.4505, -11.6651) (9.4561, -11.6692) (9.4618, -11.6733) (9.4675, -11.6775) (9.4733, -11.6817) (9.4791, -11.6859) (9.4849, -11.6901) (9.4908, -11.6943) (9.4967, -11.6985) (9.5026, -11.7027) (9.5086, -11.707) (9.5146, -11.7112) (9.5207, -11.7155) (9.5268, -11.7197) (9.5329, -11.724) (9.5391, -11.7283) (9.5453, -11.7326) (9.5516, -11.7369) (9.5578, -11.7412) (9.5642, -11.7455) (9.5705, -11.7499) (9.5769, -11.7542) (9.5833, -11.7586) (9.5898, -11.7629) (9.5963, -11.7673) (9.6028, -11.7717) (9.6094, -11.776) (9.616, -11.7804) (9.6227, -11.7848) (9.6294, -11.7892) (9.6361, -11.7936) (9.6428, -11.798) (9.6496, -11.8025) (9.6565, -11.8069) (9.6633, -11.8113) (9.6702, -11.8158) (9.6772, -11.8202) (9.6841, -11.8247) (9.6912, -11.8291) (9.6982, -11.8336) (9.7053, -11.8381) (9.7124, -11.8425) (9.7195, -11.847) (9.7267, -11.8515) (9.7339, -11.856) (9.7412, -11.8605) (9.7485, -11.865) (9.7558, -11.8695) (9.7632, -11.874) (9.7706, -11.8785) (9.778, -11.883) (9.7855, -11.8875) (9.793, -11.8921) (9.8005, -11.8966) (9.8081, -11.9011) (9.8157, -11.9056) (9.8233, -11.9102) (9.831, -11.9147) (9.8387, -11.9193) (9.8464, -11.9238) (9.8542, -11.9283) (9.862, -11.9329) (9.8699, -11.9374) (9.8777, -11.942) (9.8857, -11.9465) (9.8936, -11.9511) (9.9016, -11.9557) (9.9096, -11.9602) (9.9176, -11.9648) (9.9257, -11.9693) (9.9338, -11.9739) (9.942, -11.9785) (9.9502, -11.983) (9.9584, -11.9876) (9.9666, -11.9921) (9.9749, -11.9967) (9.9832, -12.0013) (9.9916, -12.0058) (9.9999, -12.0104) (10.0084, -12.015) (10.0168, -12.0195) (10.0253, -12.0241) (10.0338, -12.0287) (10.0423, -12.0332) (10.0509, -12.0378) (10.0595, -12.0423) (10.0682, -12.0469) (10.0768, -12.0515) (10.0855, -12.056) (10.0943, -12.0606) (10.1031, -12.0651) (10.1119, -12.0697) (10.1207, -12.0743) (10.1296, -12.0788) (10.1385, -12.0834) (10.1474, -12.0879) (10.1564, -12.0924) (10.1654, -12.097) (10.1744, -12.1015) (10.1834, -12.1061) (10.1925, -12.1106) (10.2017, -12.1151) (10.2108, -12.1197) (10.22, -12.1242) (10.2292, -12.1287) (10.2385, -12.1332) (10.2478, -12.1378) (10.2571, -12.1423) (10.2664, -12.1468) (10.2758, -12.1513) (10.2852, -12.1558) (10.2946, -12.1603) (10.3041, -12.1648) (10.3136, -12.1693) (10.3231, -12.1738) (10.3327, -12.1783) (10.3423, -12.1828) (10.35, -12.1863) (10.3558, -12.189) (10.3596, -12.1908) (10.3616, -12.1917) knots 0 0 0 0 0 0 0.00416667 0.00833333 0.0125 0.01666667 0.02083333 0.025 0.02916667 0.03333333 0.0375 0.04166667 0.04583333 0.05 0.05416667 0.05833333 0.0625 0.06666667 0.07083333 0.075 0.07916667 0.08333333 0.0875 0.09166667 0.09583333 0.1 0.10416667 0.10833333 0.1125 0.11666667 0.12083333 0.125 0.12916667 0.13333333 0.1375 0.14166667 0.14583333 0.15 0.15416667 0.15833333 0.1625 0.16666667 0.17083333 0.175 0.17916667 0.18333333 0.1875 0.19166667 0.19583333 0.2 0.20416667 0.20833333 0.2125 0.21666667 0.22083333 0.225 0.22916667 0.23333333 0.2375 0.24166667 0.24583333 0.25 0.25416667 0.25833333 0.2625 0.26666667 0.27083333 0.275 0.27916667 0.28333333 0.2875 0.29166667 0.29583333 0.3 0.30416667 0.30833333 0.3125 0.31666667 0.32083333 0.325 0.32916667 0.33333333 0.3375 0.34166667 0.34583333 0.35 0.35416667 0.35833333 0.3625 0.36666667 0.37083333 0.375 0.37916667 0.38333333 0.3875 0.39166667 0.39583333 0.4 0.40416667 0.40833333 0.4125 0.41666667 0.42083333 0.425 0.42916667 0.43333333 0.4375 0.44166667 0.44583333 0.45 0.45416667 0.45833333 0.4625 0.46666667 0.47083333 0.475 0.47916667 0.48333333 0.4875 0.49166667 0.49583333 0.5 0.50416667 0.50833333 0.5125 0.51666667 0.52083333 0.525 0.52916667 0.53333333 0.5375 0.54166667 0.54583333 0.55 0.55416667 0.55833333 0.5625 0.56666667 0.57083333 0.575 0.57916667 0.58333333 0.5875 0.59166667 0.59583333 0.6 0.60416667 0.60833333 0.6125 0.61666667 0.62083333 0.625 0.62916667 0.63333333 0.6375 0.64166667 0.64583333 0.65 0.65416667 0.65833333 0.6625 0.66666667 0.67083333 0.675 0.67916667 0.68333333 0.6875 0.69166667 0.69583333 0.7 0.70416667 0.70833333 0.7125 0.71666667 0.72083333 0.725 0.72916667 0.73333333 0.7375 0.74166667 0.74583333 0.75 0.75416667 0.75833333 0.7625 0.76666667 0.77083333 0.775 0.77916667 0.78333333 0.7875 0.79166667 0.79583333 0.8 0.80416667 0.80833333 0.8125 0.81666667 0.82083333 0.825 0.82916667 0.83333333 0.8375 0.84166667 0.84583333 0.85 0.85416667 0.85833333 0.8625 0.86666667 0.87083333 0.875 0.87916667 0.88333333 0.8875 0.89166667 0.89583333 0.9 0.90416667 0.90833333 0.9125 0.91666667 0.92083333 0.925 0.92916667 0.93333333 0.9375 0.94166667 0.94583333 0.95 0.95416667 0.95833333 0.9625 0.96666667 0.97083333 0.975 0.97916667 0.98333333 0.9875 0.99166667 0.99583333 1 1 1 1 1 1
  line L107 (11.5731, 7.4247) -> (12.223, 7.8417)
  line L108 (-12.223, -7.8417) -> (-12.2236, -7.8421)
  line L109 (-12.9026, -6.6646) -> (-12.2165, -6.3102)
  line L110 (10.326, -10.2121) -> (10.3255, -10.2117)
  line L111 (14.3558, 2.1922) -> (14.3564, 2.1923)
  circle A65 centre (7.0711, 7.0711) radius 1.7
  line L112 (12.223, 7.8417) -> (12.2236, 7.8421)
  spline S55 degree 5 poles (-14.4246, -6.9233) (-14.4224, -6.9232) (-14.4182, -6.9232) (-14.4118, -6.9231) (-14.4033, -6.9229) (-14.3927, -6.9227) (-14.3822, -6.9225) (-14.3716, -6.9223) (-14.3611, -6.9221) (-14.3507, -6.9218) (-14.3402, -6.9215) (-14.3298, -6.9212) (-14.3194, -6.9209) (-14.309, -6.9206) (-14.2987, -6.9203) (-14.2883, -6.9199) (-14.2781, -6.9195) (-14.2678, -6.9192) (-14.2576, -6.9188) (-14.2474, -6.9183) (-14.2372, -6.9179) (-14.227, -6.9175) (-14.2169, -6.917) (-14.2068, -6.9165) (-14.1967, -6.916) (-14.1867, -6.9155) (-14.1767, -6.915) (-14.1667, -6.9145) (-14.1568, -6.9139) (-14.1468, -6.9134) (-14.1369, -6.9128) (-14.1271, -6.9122) (-14.1172, -6.9116) (-14.1074, -6.9109) (-14.0976, -6.9103) (-14.0879, -6.9097) (-14.0782, -6.909) (-14.0685, -6.9083) (-14.0588, -6.9076) (-14.0492, -6.9069) (-14.0396, -6.9062) (-14.03, -6.9055) (-14.0205, -6.9047) (-14.011, -6.9039) (-14.0015, -6.9032) (-13.992, -6.9024) (-13.9826, -6.9016) (-13.9732, -6.9008) (-13.9639, -6.8999) (-13.9545, -6.8991) (-13.9452, -6.8982) (-13.936, -6.8974) (-13.9267, -6.8965) (-13.9175, -6.8956) (-13.9083, -6.8947) (-13.8992, -6.8938) (-13.8901, -6.8929) (-13.881, -6.8919) (-13.872, -6.891) (-13.8629, -6.89) (-13.854, -6.889) (-13.845, -6.888) (-13.8361, -6.887) (-13.8272, -6.886) (-13.8184, -6.885) (-13.8095, -6.884) (-13.8007, -6.8829) (-13.792, -6.8818) (-13.7833, -6.8808) (-13.7746, -6.8797) (-13.7659, -6.8786) (-13.7573, -6.8775) (-13.7487, -6.8764) (-13.7401, -6.8753) (-13.7316, -6.8741) (-13.7231, -6.873) (-13.7147, -6.8718) (-13.7063, -6.8707) (-13.6979, -6.8695) (-13.6895, -6.8683) (-13.6812, -6.8671) (-13.6729, -6.8659) (-13.6647, -6.8647) (-13.6564, -6.8635) (-13.6483, -6.8623) (-13.6401, -6.861) (-13.632, -6.8598) (-13.6239, -6.8585) (-13.6159, -6.8572) (-13.6079, -6.856) (-13.5999, -6.8547) (-13.592, -6.8534) (-13.5841, -6.8521) (-13.5762, -6.8508) (-13.5684, -6.8494) (-13.5606, -6.8481) (-13.5528, -6.8468) (-13.5451, -6.8454) (-13.5375, -6.8441) (-13.5298, -6.8427) (-13.5222, -6.8414) (-13.5146, -6.84) (-13.5071, -6.8386) (-13.4996, -6.8372) (-13.4922, -6.8358) (-13.4847, -6.8344) (-13.4773, -6.833) (-13.47, -6.8316) (-13.4627, -6.8302) (-13.4554, -6.8288) (-13.4482, -6.8273) (-13.441, -6.8259) (-13.4339, -6.8244) (-13.4267, -6.823) (-13.4197, -6.8215) (-13.4126, -6.8201) (-13.4056, -6.8186) (-13.3987, -6.8171) (-13.3918, -6.8157) (-13.3849, -6.8142) (-13.378, -6.8127) (-13.3712, -6.8112) (-13.3645, -6.8097) (-13.3578, -6.8082) (-13.3511, -6.8067) (-13.3445, -6.8052) (-13.3379, -6.8037) (-13.3313, -6.8022) (-13.3248, -6.8007) (-13.3183, -6.7992) (-13.3119, -6.7976) (-13.3055, -6.7961) (-13.2991, -6.7946) (-13.2928, -6.7931) (-13.2866, -6.7915) (-13.2804, -6.79) (-13.2742, -6.7885) (-13.268, -6.7869) (-13.2619, -6.7854) (-13.2559, -6.7839) (-13.2499, -6.7823) (-13.2439, -6.7808) (-13.238, -6.7792) (-13.2321, -6.7777) (-13.2263, -6.7761) (-13.2205, -6.7746) (-13.2147, -6.7731) (-13.209, -6.7715) (-13.2034, -6.77) (-13.1978, -6.7684) (-13.1922, -6.7669) (-13.1867, -6.7653) (-13.1812, -6.7638) (-13.1758, -6.7623) (-13.1704, -6.7607) (-13.165, -6.7592) (-13.1597, -6.7577) (-13.1545, -6.7561) (-13.1493, -6.7546) (-13.1441, -6.7531) (-13.139, -6.7516) (-13.1339, -6.75) (-13.1289, -6.7485) (-13.124, -6.747) (-13.119, -6.7455) (-13.1142, -6.744) (-13.1093, -6.7425) (-13.1046, -6.741) (-13.0998, -6.7395) (-13.0951, -6.738) (-13.0905, -6.7366) (-13.0859, -6.7351) (-13.0814, -6.7336) (-13.0769, -6.7321) (-13.0725, -6.7307) (-13.0681, -6.7292) (-13.0638, -6.7278) (-13.0595, -6.7264) (-13.0552, -6.7249) (-13.0511, -6.7235) (-13.0469, -6.7221) (-13.0429, -6.7207) (-13.0388, -6.7193) (-13.0349, -6.7179) (-13.0309, -6.7165) (-13.0271, -6.7152) (-13.0232, -6.7138) (-13.0195, -6.7125) (-13.0158, -6.7111) (-13.0121, -6.7098) (-13.0085, -6.7085) (-13.005, -6.7072) (-13.0015, -6.7059) (-12.998, -6.7046) (-12.9946, -6.7033) (-12.9913, -6.7021) (-12.988, -6.7008) (-12.9848, -6.6996) (-12.9816, -6.6984) (-12.9785, -6.6972) (-12.9755, -6.696) (-12.9725, -6.6948) (-12.9695, -6.6937) (-12.9667, -6.6925) (-12.9638, -6.6914) (-12.9611, -6.6903) (-12.9584, -6.6892) (-12.9557, -6.6881) (-12.9531, -6.6871) (-12.9506, -6.686) (-12.9482, -6.685) (-12.9457, -6.684) (-12.9434, -6.683) (-12.9411, -6.6821) (-12.9389, -6.6811) (-12.9367, -6.6802) (-12.9346, -6.6793) (-12.9326, -6.6784) (-12.9306, -6.6775) (-12.9287, -6.6767) (-12.9269, -6.6759) (-12.9251, -6.6751) (-12.9234, -6.6743) (-12.9217, -6.6736) (-12.9201, -6.6729) (-12.9186, -6.6722) (-12.9171, -6.6715) (-12.9157, -6.6709) (-12.9144, -6.6703) (-12.9132, -6.6697) (-12.912, -6.6691) (-12.9108, -6.6686) (-12.9098, -6.6681) (-12.9088, -6.6676) (-12.9079, -6.6672) (-12.9071, -6.6668) (-12.9063, -6.6664) (-12.9056, -6.6661) (-12.905, -6.6658) (-12.9044, -6.6655) (-12.9039, -6.6652) (-12.9036, -6.6651) (-12.9034, -6.665) (-12.9033, -6.6649) (-12.9032, -6.6649) knots -1 -1 -1 -1 -1 -1 -0.99583333 -0.99166667 -0.9875 -0.98333333 -0.97916667 -0.975 -0.97083333 -0.96666667 -0.9625 -0.95833333 -0.95416667 -0.95 -0.94583333 -0.94166667 -0.9375 -0.93333333 -0.92916667 -0.925 -0.92083333 -0.91666667 -0.9125 -0.90833333 -0.90416667 -0.9 -0.89583333 -0.89166667 -0.8875 -0.88333333 -0.87916667 -0.875 -0.87083333 -0.86666667 -0.8625 -0.85833333 -0.85416667 -0.85 -0.84583333 -0.84166667 -0.8375 -0.83333333 -0.82916667 -0.825 -0.82083333 -0.81666667 -0.8125 -0.80833333 -0.80416667 -0.8 -0.79583333 -0.79166667 -0.7875 -0.78333333 -0.77916667 -0.775 -0.77083333 -0.76666667 -0.7625 -0.75833333 -0.75416667 -0.75 -0.74583333 -0.74166667 -0.7375 -0.73333333 -0.72916667 -0.725 -0.72083333 -0.71666667 -0.7125 -0.70833333 -0.70416667 -0.7 -0.69583333 -0.69166667 -0.6875 -0.68333333 -0.67916667 -0.675 -0.67083333 -0.66666667 -0.6625 -0.65833333 -0.65416667 -0.65 -0.64583333 -0.64166667 -0.6375 -0.63333333 -0.62916667 -0.625 -0.62083333 -0.61666667 -0.6125 -0.60833333 -0.60416667 -0.6 -0.59583333 -0.59166667 -0.5875 -0.58333333 -0.57916667 -0.575 -0.57083333 -0.56666667 -0.5625 -0.55833333 -0.55416667 -0.55 -0.54583333 -0.54166667 -0.5375 -0.53333333 -0.52916667 -0.525 -0.52083333 -0.51666667 -0.5125 -0.50833333 -0.50416667 -0.5 -0.49583333 -0.49166667 -0.4875 -0.48333333 -0.47916667 -0.475 -0.47083333 -0.46666667 -0.4625 -0.45833333 -0.45416667 -0.45 -0.44583333 -0.44166667 -0.4375 -0.43333333 -0.42916667 -0.425 -0.42083333 -0.41666667 -0.4125 -0.40833333 -0.40416667 -0.4 -0.39583333 -0.39166667 -0.3875 -0.38333333 -0.37916667 -0.375 -0.37083333 -0.36666667 -0.3625 -0.35833333 -0.35416667 -0.35 -0.34583333 -0.34166667 -0.3375 -0.33333333 -0.32916667 -0.325 -0.32083333 -0.31666667 -0.3125 -0.30833333 -0.30416667 -0.3 -0.29583333 -0.29166667 -0.2875 -0.28333333 -0.27916667 -0.275 -0.27083333 -0.26666667 -0.2625 -0.25833333 -0.25416667 -0.25 -0.24583333 -0.24166667 -0.2375 -0.23333333 -0.22916667 -0.225 -0.22083333 -0.21666667 -0.2125 -0.20833333 -0.20416667 -0.2 -0.19583333 -0.19166667 -0.1875 -0.18333333 -0.17916667 -0.175 -0.17083333 -0.16666667 -0.1625 -0.15833333 -0.15416667 -0.15 -0.14583333 -0.14166667 -0.1375 -0.13333333 -0.12916667 -0.125 -0.12083333 -0.11666667 -0.1125 -0.10833333 -0.10416667 -0.1 -0.09583333 -0.09166667 -0.0875 -0.08333333 -0.07916667 -0.075 -0.07083333 -0.06666667 -0.0625 -0.05833333 -0.05416667 -0.05 -0.04583333 -0.04166667 -0.0375 -0.03333333 -0.02916667 -0.025 -0.02083333 -0.01666667 -0.0125 -0.00833333 -0.00416667 0 0 0 0 0 0